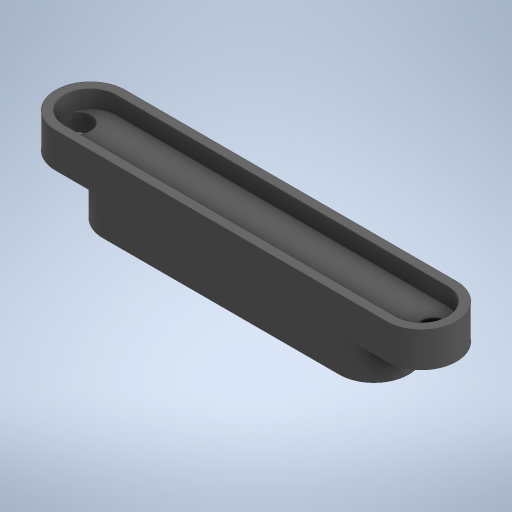
# Autodesk Inventor part: Connector1
Saved by Autodesk Inventor 2023 (Build 270158000, 158)
## iProperties
Created: 2024-03-26
Part Number: Connector1
Material: Generic
Document SubType Name: Modeling
Designer: noname
Density: 1 g/cm^3
Appearance: Default
Author: noname
Autodesk Inventor part; units mm, degrees
ref_plane "YZ Plane" through (0, 0, 0) normal (1, 0, 0) x (0, 1, 0)
ref_plane "XZ Plane" through (0, 0, 0) normal (0, 1, 0) x (-1, 0, 0)
ref_plane "XY Plane" through (0, 0, 0) normal (0, 0, 1) x (1, 0, 0)
sketch "Sketch1" plane through (0, 0, 0) normal (0, 1, 0) x (-1, 0, 0)
  line L0 (-16.7648, -6.8244) -> (19.5108, -6.8244) construction
  line L1 (19.5108, -6.8244) -> (19.5108, -28.8158) construction
  line L2 (19.5108, -28.8158) -> (-16.7648, -28.8158) construction
  line L3 (-16.7648, -28.8158) -> (-16.7648, -6.8244) construction
  line L4 (6.77, 0) -> (-6.77, 0) construction
  line L5 (6.77, 2) -> (-6.77, 2)
  line L6 (-6.77, -2) -> (6.77, -2)
  arc A0 (6.77, -2) -> (6.77, 2) centre (6.77, 0) ccw
  arc A1 (-6.77, 2) -> (-6.77, -2) centre (-6.77, 0) ccw
  point P0 (0, 0)
  point P1 (-8.77, 0)
  point P2 (8.77, 0)
  dimension "d11" = 17.54
  dimension "d18" = 4
  constraints: 8 end point, 6 point on circle, 4 tangent, 2 centre point, 1 horizontal, 1 midpoint, 1 parallel, 2 other
  measures "d11" distance of point (-8.77, 0) point (8.77, 0)
  measures "d18" distance between parallel lines of L5 L6
extrude "Extrusion1" add sketch "Sketch1" along normal blind 2
sketch "Sketch2" plane through (0, 2, 0) normal (0, 1, 0) x (1, 0, 0)
  arc A0 (6.77, -2) -> (6.77, 2) centre (6.77, 0) ccw projected
  line L0 (6.77, 2) -> (-6.77, 2) projected
  arc A1 (-6.77, 2) -> (-6.77, -2) centre (-6.77, 0) ccw projected
  line L1 (-6.77, -2) -> (6.77, -2) projected
  line L2 (-9.5, 0) -> (9.5, 0) construction
  line L3 (-9.5, -2) -> (9.5, -2)
  line L4 (9.5, 2) -> (-9.5, 2)
  arc A2 (-9.5, 2) -> (-9.5, -2) centre (-9.5, 0) ccw
  arc A3 (9.5, -2) -> (9.5, 2) centre (9.5, 0) ccw
  circle A4 centre (-10.22, 0) radius 0.75
  line L5 (0, -2) -> (0, 2)
  circle A5 centre (10.22, 0) radius 0.75
  point P0 (0, 0)
  point P1 (11.5, 0)
  point P2 (-11.5, 0)
  point P3 (0, 0)
  point P4 (-6.77, -2)
  point P5 (6.77, -2)
  dimension "d23" = 4
  dimension "d24" = 23
  dimension "d25" = 1.5
  dimension "d26" = 20.44
  constraints: 10 end point, 6 point on circle, 4 centre point, 4 midpoint, 4 tangent, 1 horizontal, 1 horizontal alignment, 1 parallel, 1 symmetric about line, 1 other
  measures "d23" distance between parallel lines of L3 L4
  measures "d24" distance of point (11.5, 0) point (-11.5, 0)
  measures "d25" diameter of A4
  measures "d26" distance of A5.centre A4.centre
extrude "Extrusion2" add sketch "Sketch2" along normal blind 1
sketch "Sketch3" plane through (0, 3, 0) normal (0, 1, 0) x (1, 0, 0)
  line L0 (9.5, 2) -> (-9.5, 2) projected
  arc A0 (-9.5, 2) -> (-9.5, -2) centre (-9.5, 0) ccw projected
  line L1 (-9.5, -2) -> (9.5, -2) projected
  arc A1 (9.5, -2) -> (9.5, 2) centre (9.5, 0) ccw projected
  circle A2 centre (-10.22, 0) radius 0.75 projected
  circle A3 centre (10.22, 0) radius 0.75 projected
  line L2 (-9.5, 1.5) -> (9.5, 1.5)
  arc A4 (9.5, -1.5) -> (9.5, 1.5) centre (9.5, 0) ccw
  line L3 (9.5, -1.5) -> (-9.5, -1.5)
  arc A5 (-9.5, 1.5) -> (-9.5, -1.5) centre (-9.5, 0) ccw
  point P0 (0, 0)
  dimension "d29" = 0.5
  constraints: 4 end point, 4 point on circle, 2 centre point, 3 other
  measures "d29" distance between parallel lines of L2 L0
extrude "Extrusion3" add sketch "Sketch3" along normal blind 1 contours A1 L1 A0 L0
sketch "Sketch4" plane through (0, 0, 0) normal (0, -1, 0) x (1, 0, 0)
  circle A0 centre (-3.81, 0) radius 0.755
  circle A1 centre (-1.27, 0) radius 0.755
  line L0 (-6.77, 2) -> (6.77, 2) projected
  line L1 (0, 2) -> (0, -2)
  line L2 (6.77, -2) -> (-6.77, -2) projected
  circle A2 centre (3.81, 0) radius 0.755
  circle A3 centre (1.27, 0) radius 0.755
  point P0 (0, 0)
  dimension "d32" = 2.54
  dimension "d33" = 7.62
  dimension "d34" = 1.51
  constraints: 4 centre point, 2 end point, 2 midpoint, 2 symmetric about line, 1 equal radius, 2 other
  measures "d32" distance of A3.centre A1.centre
  measures "d33" distance of A0.centre A2.centre
  measures "d34" diameter of A2
extrude "Extrusion4" cut sketch "Sketch4" against normal blind 1
sketch "Sketch5" plane through (-3.81, 1, 0) normal (0, -1, 0) x (1, 0, 0)
  circle A0 centre (0, 0) radius 0.755 projected
  circle A1 centre (2.54, 0) radius 0.755 projected
  circle A2 centre (5.08, 0) radius 0.755 projected
  circle A3 centre (7.62, 0) radius 0.755 projected
  circle A4 centre (0, 0) radius 0.755 projected
  circle A5 centre (0, 0) radius 0.45
  circle A6 centre (2.54, 0) radius 0.45
  circle A7 centre (5.08, 0) radius 0.45
  circle A8 centre (7.62, 0) radius 0.45
  point P0 (3.81, 0)
  dimension "d37" = 0.9
  constraints: 4 centre point, 4 coincident, 3 equal radius
  measures "d37" diameter of A6
extrude "Extrusion5" add sketch "Sketch5" along normal blind 2 contours A5 | A6 | A7 | A8
fillet "Fillet1" radius 0.45 4 edges at (-4.26, -1, 0) (-1.72, -1, 0) (0.82, -1, 0) (3.36, -1, 0)
sketch "Sketch6" plane through (0, 0, 0) normal (0, -1, 0) x (1, 0, 0)
  circle A0 centre (1.27, 0) radius 0.755 projected
  circle A1 centre (-1.27, 0) radius 0.755 projected
  circle A2 centre (3.81, 0) radius 0.755 projected
  circle A3 centre (-3.81, 0) radius 0.755 projected
  arc A4 (6.77, -2) -> (6.77, 2) centre (6.77, 0) ccw projected
  line L0 (-6.77, 2) -> (6.77, 2) projected
  arc A5 (-6.77, 2) -> (-6.77, -2) centre (-6.77, 0) ccw projected
  line L1 (6.77, -2) -> (-6.77, -2) projected
  circle A6 centre (-6.77, 0) radius 1.5
  circle A7 centre (6.77, 0) radius 1.5
  point P0 (0, 0)
  dimension "d41" = 3
  constraints: 2 centre point, 2 coincident, 1 equal radius
  measures "d41" diameter of A6
extrude "Extrusion6" cut sketch "Sketch6" against normal blind 0.1 contours A6 | A7
body "Solid1"
